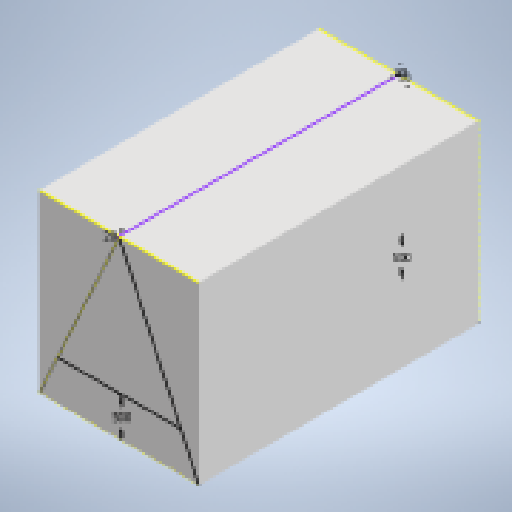
# Autodesk Inventor part: SzofiHinta
Saved by Autodesk Inventor 2025.2 (Build 292293000, 293)
## iProperties
Created: 2025-02-26
Part Number: SzofiHinta
Material: Generic
Document SubType Name: Modeling
Designer: MB
Density: 1 g/cm^3
Appearance: Default
Author: MB
Autodesk Inventor part; units mm, degrees
ref_plane "YZ Plane" through (0, 0, 0) normal (1, 0, 0) x (0, 1, 0)
ref_plane "XZ Plane" through (0, 0, 0) normal (0, 1, 0) x (-1, 0, 0)
ref_plane "XY Plane" through (0, 0, 0) normal (0, 0, 1) x (1, 0, 0)
sketch "Sketch2" plane through (0, 0, 0) normal (0, 1, 0) x (-1, 0, 0)
  line L0 (0, 0) -> (1800, 0)
  line L1 (1800, 0) -> (1800, -3500)
  line L2 (1800, -3500) -> (0, -3500)
  line L3 (0, -3500) -> (0, 0)
  dimension "Base_Width" = 1800
  dimension "Base_Length" = 3500
  constraints: 8 end point, 2 parallel, 1 horizontal, 1 perpendicular
  measures "Base_Width" distance of L1.end L2.end
  measures "Base_Length" distance of L0.end L1.end
extrude "Extrusion1" add sketch "Sketch2" along normal blind 2200
sketch "Sketch4" plane through (0, 0, -3500) normal (0, 0, -1) x (-1, 0, 0)
  line L0 (0, 0) -> (1800, 0) construction
  line L1 (0, 0) -> (1800, 0) construction
  line L2 (1800, 0) -> (1800, 2200) construction
  line L3 (0, 2200) -> (1800, 2200) construction
  line L4 (0, 0) -> (0, 2200) construction
  line L5 (0, 0) -> (900, 2200)
  line L6 (1800, 0) -> (896.2137, 2190.7445)
  line L7 (0, 2200) -> (1800, 2200) projected
  line L8 (204.5455, 500) -> (1593.7262, 500)
  dimension "d10" = 10
  dimension "d12" = 500
  constraints: 6 end point, 3 point on line, 2 midpoint, 1 horizontal
  measures "d10" distance of L6.end point (900, 2200)
  measures "d12" distance between parallel lines of L0 L8
sketch "Sketch5" plane through (0, 2200, 0) normal (0, 1, 0) x (1, 0, 0)
  line L0 (-1800, 0) -> (0, 0) construction
  line L1 (0, 3500) -> (-1800, 3500) construction
  line L2 (0, 3500) -> (-1800, 3500) construction
  line L3 (-1800, 3500) -> (-1800, 0) construction
  line L4 (-1800, 0) -> (0, 0) construction
  line L5 (0, 0) -> (0, 3500) construction
  line L6 (-900, -20) -> (-900, 3520)
  dimension "d17" = 20
  dimension "d18" = 20
  dimension "d19" = 900
  constraints: 2 end point, 1 perpendicular
  measures "d17" distance from line of L1 L6.end
  measures "d18" distance from line of L0 L6.start
  measures "d19" distance between parallel lines of L5 L6
sketch "Sketch6" plane through (-1800, 0, 0) normal (0, 0, 1) x (1, 0, 0)
  line L0 (1800, 0) -> (900, 2200) construction
  line L1 (0, 0) -> (903.7863, 2190.7445) construction
  line L2 (1800, 0) -> (0, 0) construction
  line L3 (0, 0) -> (903.7863, 2190.7445)
  line L4 (900, 2200) -> (1800, 0)
  line L5 (206.2738, 500) -> (1595.4545, 500)
  point P0 (900.8642, 500)
  dimension "d11" = 500
  constraints: 6 end point, 2 collinear, 2 point on line, 1 horizontal, 1 midpoint
  measures "d11" distance from line of L2 point (900.864, 500)
equation "\"d19\" = 0.5 * Base_Width"
body "Solid1"
